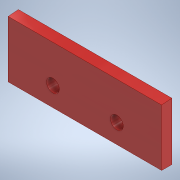
# Autodesk Inventor part: Lower blade
Saved by Autodesk Inventor 2020.3 (Build 243373000, 373)
## iProperties
Created: 2021-06-11
Part Number: Lower blade
Material: Steel, Mild
Document SubType Name: Modeling
Designer: User
Density: 7.85 g/cm^3
Appearance: Orange-Red
Mass: 324.087 g
Surface Area: 135.187 cm^2
Volume: 41.285 cm^3
Author: User
Autodesk Inventor part; units mm, degrees
ref_plane "YZ Plane" through (0, 0, 0) normal (1, 0, 0) x (0, 1, 0)
ref_plane "XZ Plane" through (0, 0, 0) normal (0, 1, 0) x (-1, 0, 0)
ref_plane "XY Plane" through (0, 0, 0) normal (0, 0, 1) x (1, 0, 0)
sketch "Sketch1" plane through (0, 0, 0) normal (0, 0, 1) x (1, 0, 0)
  line L0 (-60, -22.5) -> (60, -22.5)
  line L1 (60, -22.5) -> (60, 22.5)
  line L2 (60, 22.5) -> (-60, 22.5)
  line L3 (-60, 22.5) -> (-60, -22.5)
  line L4 (-60, -22.5) -> (60, 22.5) construction
  line L5 (60, -22.5) -> (-60, 22.5) construction
  circle A0 centre (-25, -7.5) radius 5
  circle A1 centre (25, -7.5) radius 5
  point P0 (0, 0)
  dimension "d0" = 120
  dimension "d1" = 45
  dimension "d2" = 10
  dimension "d3" = 10
  dimension "d4" = 35
  dimension "d5" = 35
  dimension "d6" = 15
  dimension "d7" = 15
  constraints: 12 end point, 2 centre point, 2 midpoint, 2 parallel, 1 horizontal, 1 perpendicular
  measures "d0" distance of L1.end L2.end
  measures "d1" distance of L0.end L1.end
  measures "d2" diameter of A1
  measures "d3" diameter of A0
  measures "d4" distance from line of L1 A1.centre
  measures "d5" distance from line of L3 A0.centre
  measures "d6" distance from line of L0 A0.centre
  measures "d7" distance from line of L0 A1.centre
extrude "Extrusion1" add sketch "Sketch1" along normal blind 7.9375
chamfer "Chamfer1" distance 7.9375 angle 5 1 edges at (0, 22.5, 7.9375) measured on face at (20, 22.5, 2.6458)
body "Solid1"
